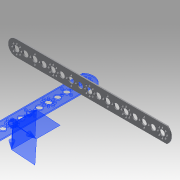
# Autodesk Inventor part: Tetrix Max Flat 288mm
Saved by Autodesk Inventor 2016 (Build 200138000, 138)
## iProperties
Created: 2015-10-23
Part Number: Tetrix Max Flat 288mm
Material: Generic
Document SubType Name: Modeling
Designer: Delta
Density: 1 g/cm^3
Appearance: Default
Mass: 11.1302 g
Surface Area: 145.248 cm^2
Volume: 11.1302 cm^3
Author: Delta
Autodesk Inventor part; units mm, degrees
ref_plane "YZ Plane" through (0, 0, 0) normal (1, 0, 0) x (0, 1, 0)
ref_plane "XZ Plane" through (0, 0, 0) normal (0, 1, 0) x (-1, 0, 0)
ref_plane "XY Plane" through (0, 0, 0) normal (0, 0, 1) x (1, 0, 0)
sketch "Sketch1" plane through (0, 0, 0) normal (0, 0, 1) x (1, 0, 0)
  line L0 (0, 0) -> (288, 0)
  line L1 (288, 0) -> (288, 27)
  line L2 (288, 27) -> (0, 27)
  line L3 (0, 27) -> (0, 0)
  dimension "d0" = 288
  dimension "d1" = 27
  constraints: 8 end point, 2 parallel, 1 horizontal, 1 perpendicular
  measures "d0" distance of L2.end L1.end
  measures "d1" distance of L1.end L0.end
extrude "Extrusion1" add sketch "Sketch1" along normal blind 2.04
sketch "Sketch2" plane through (0, 0, 2.04) normal (0, 0, 1) x (1, 0, 0)
  line L0 (0, 27) -> (0, 0) projected
  line L1 (0, 0) -> (0, 13.5001)
  line L2 (0, 13.5001) -> (14.275, 13.5001)
  line L3 (0, 13.5001) -> (14.275, 13.5001) construction
  circle A0 centre (14.275, 13.5001) radius 4.875
  line L4 (14.275, 13.5001) -> (16.815, 13.5001)
  circle A1 centre (30.005, 13.5001) radius 4.875
  circle A2 centre (45.735, 13.5001) radius 4.875
  circle A3 centre (61.465, 13.5001) radius 4.875
  circle A4 centre (77.195, 13.5001) radius 4.875
  circle A5 centre (92.925, 13.5001) radius 4.875
  circle A6 centre (108.655, 13.5001) radius 4.875
  circle A7 centre (124.385, 13.5001) radius 4.875
  circle A8 centre (140.115, 13.5001) radius 4.875
  circle A9 centre (155.845, 13.5001) radius 4.875
  circle A10 centre (171.575, 13.5001) radius 4.875
  circle A11 centre (187.305, 13.5001) radius 4.875
  circle A12 centre (203.035, 13.5001) radius 4.875
  circle A13 centre (218.765, 13.5001) radius 4.875
  circle A14 centre (234.495, 13.5001) radius 4.875
  circle A15 centre (250.225, 13.5001) radius 4.875
  circle A16 centre (265.955, 13.5001) radius 4.875
  dimension "d4" = 13.5001
  dimension "d5" = 14.275
  dimension "d6" = 0
  dimension "d7" = 9.75
  dimension "d8" = 2.54
  dimension "d13" = 15.73
  constraints: 17 centre point, 8 end point, 4 horizontal, 1 coincident, 1 collinear, 1 point on line, 48 other
  measures "d4" distance of L0.end L1.end
  measures "d5" distance of L1.end L2.end
  measures "d6" distance between parallel lines of L2 L3
  measures "d7" diameter of A0
  measures "d8" distance of L4.start L4.end
  measures "d13" distance of L4.start A1.centre
extrude "Extrusion2" cut sketch "Sketch2" against normal blind 2.04
fillet "Fillet1" radius 13.5 4 edges at (0, 27, 1.02) (0, 0, 1.02) (288, 27, 1.02) (288, 0, 1.02)
sketch "Sketch3" plane through (0, 0, 2.04) normal (0, 0, 1) x (1, 0, 0)
  line L0 (13.5, 0) -> (274.5, 0) projected
  line L1 (0, 13.362) -> (0, 13.208) projected
  circle A0 centre (14.275, 13.5001) radius 4.875 projected
  line L2 (14.275, 8.6251) -> (14.275, 18.3751)
  line L3 (9.4, 13.5001) -> (19.15, 13.5001)
  line L4 (14.275, 13.5001) -> (14.275, 21.3651)
  line L5 (274.5, 27) -> (13.5, 27) projected
  line L6 (10.8279, 10.053) -> (17.7221, 16.9472)
  line L7 (14.275, 8.6251) -> (14.275, 18.3751)
  line L8 (17.7221, 10.053) -> (10.8279, 16.9472)
  line L9 (19.15, 13.5001) -> (9.4, 13.5001)
  line L10 (17.7221, 16.9472) -> (10.8279, 10.053)
  line L11 (14.275, 18.3751) -> (14.275, 8.6251)
  line L12 (10.8279, 16.9472) -> (17.7221, 10.053)
  point P0 (0, 0)
  point P1 (8.7136, 19.0615)
  point P2 (6.41, 13.5001)
  point P3 (8.7136, 7.9387)
  point P4 (14.275, 5.6351)
  point P5 (19.8364, 7.9387)
  point P6 (22.14, 13.5001)
  point P7 (19.8364, 19.0615)
  dimension "d30" = 360
  dimension "d39" = 7.865
  constraints: 20 end point, 4 point on circle, 3 coincident, 1 horizontal, 1 perpendicular, 1 vertical, 39 other
  measures "d39" distance of L4.start L4.end
hole "Hole1" at (14.275, 21.3651, 2.04) at (8.7136, 19.0615, 2.04) at (6.41, 13.5001, 2.04) at (8.7136, 7.9387, 2.04) at (14.275, 5.6351, 2.04) at (19.8364, 7.9387, 2.04) at (22.14, 13.5001, 2.04) at (19.8364, 19.0615, 2.04) direction (0, 0, -1) diameter 3.73 end through all
pattern_linear "Rectangular Pattern1" count 5 spacing 62.92 along (1, 0, 0) of "Hole1"
sketch "Sketch4" plane through (0, 0, 2.04) normal (0, 0, 1) x (1, 0, 0)
  line L0 (45.5847, 13.5001) -> (45.5847, 21.3651)
  circle A0 centre (30.005, 13.5001) radius 4.875 projected
  line L1 (30.005, 13.5001) -> (35.5959, 13.5001)
  line L2 (30.005, 13.5001) -> (35.5959, 13.5001) construction
  line L3 (30.005, 13.5001) -> (45.5847, 13.5001)
  point P0 (0, 0)
  point P1 (37.7197, 13.5001)
  point P2 (45.5847, 5.6351)
  point P3 (53.4497, 13.5001)
  point P4 (116.3697, 13.5001)
  point P5 (108.5047, 5.6351)
  point P6 (100.6397, 13.5001)
  point P7 (108.5047, 21.3651)
  point P8 (179.2897, 13.5001)
  point P9 (171.4247, 5.6351)
  point P10 (163.5597, 13.5001)
  point P11 (171.4247, 21.3651)
  point P12 (242.2097, 13.5001)
  point P13 (234.3447, 5.6351)
  point P14 (226.4797, 13.5001)
  point P15 (234.3447, 21.3651)
  dimension "d43" = 7.865
  dimension "d46" = 360
  dimension "d48" = 0
  dimension "d49" = 15.5797
  dimension "d52" = 62.92
  constraints: 8 end point, 3 horizontal, 1 coincident, 1 collinear, 1 vertical, 17 other
  measures "d43" distance of L0.start L0.end
  measures "d48" distance between parallel lines of L1 L2
  measures "d49" distance of L1.start L0.start
  measures "d52" distance of point (53.45, 13.5) point (116.37, 13.5)
hole "Hole2" at (45.5847, 5.6351, 2.04) at (53.4497, 13.5001, 2.04) at (45.5847, 21.3651, 2.04) at (37.7197, 13.5001, 2.04) at (100.6397, 13.5001, 2.04) at (108.5047, 5.6351, 2.04) at (116.3697, 13.5001, 2.04) at (108.5047, 21.3651, 2.04) at (171.4247, 21.3651, 2.04) at (179.2897, 13.5001, 2.04) at (171.4247, 5.6351, 2.04) at (163.5597, 13.5001, 2.04) at (234.3447, 5.6351, 2.04) at (226.4797, 13.5001, 2.04) at (242.2097, 13.5001, 2.04) at (234.3447, 21.3651, 2.04) direction (0, 0, -1) diameter 3.73 end through all
sketch "Sketch5" plane through (0, 0, 0) normal (0, 0, -1) x (-1, 0, 0)
  arc A0 (-274.5, 27) -> (-274.5, 0) centre (-274.5, 13.5) ccw projected
  arc A1 (-274.5, 27) -> (-274.5, 0) centre (-263.4244, 13.5) ccw
  point P0 (0, 0)
  constraints: 2 point on circle, 1 centre point
extrude "Extrusion3" cut sketch "Sketch5" against normal through all
body "Solid1"
